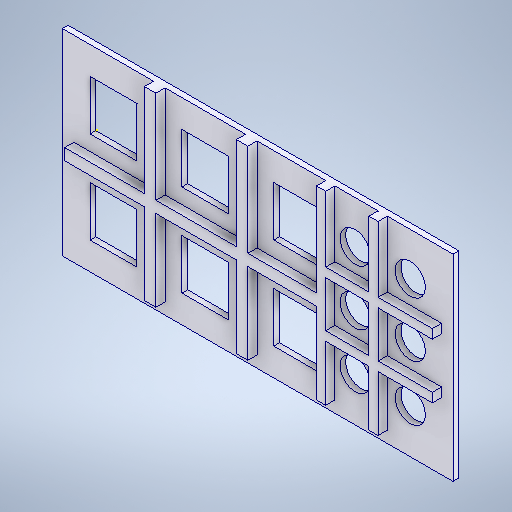
# Autodesk Inventor part: faceplate
Saved by Autodesk Inventor 2025 (Build 290162000, 162)
## iProperties
Created: 2024-08-10
Part Number: faceplate
Material: Generic
Document SubType Name: Modeling
Designer: ethan
Density: 1 g/cm^3
Appearance: Cool White
Author: ethan
Autodesk Inventor part; units mm, degrees
ref_plane "YZ Plane" through (0, 0, 0) normal (1, 0, 0) x (0, 1, 0)
ref_plane "XZ Plane" through (0, 0, 0) normal (0, 1, 0) x (-1, 0, 0)
ref_plane "XY Plane" through (0, 0, 0) normal (0, 0, 1) x (1, 0, 0)
sketch "Sketch1" plane through (0, 0, 0) normal (0, 0, 1) x (1, 0, 0)
  point P0 (0, 0)
sketch "Sketch2" plane through (0, 0, 0) normal (0, 0, 1) x (1, 0, 0)
  line L0 (0, 0) -> (20.4, 0)
  line L1 (20.4, 0) -> (20.4, 21.7)
  line L2 (20.4, 21.7) -> (0, 21.7)
  line L3 (0, 21.7) -> (0, 0)
  line L4 (40, 0) -> (60.4, 0)
  line L5 (60.4, 0) -> (60.4, 21.7)
  line L6 (60.4, 21.7) -> (40, 21.7)
  line L7 (40, 21.7) -> (40, 0)
  line L8 (80, 0) -> (100.4, 0)
  line L9 (100.4, 0) -> (100.4, 21.7)
  line L10 (100.4, 21.7) -> (80, 21.7)
  line L11 (80, 21.7) -> (80, 0)
  line L12 (0, -40) -> (20.4, -40)
  line L13 (20.4, -40) -> (20.4, -18.3)
  line L14 (20.4, -18.3) -> (0, -18.3)
  line L15 (0, -18.3) -> (0, -40)
  line L16 (40, -40) -> (60.4, -40)
  line L17 (60.4, -40) -> (60.4, -18.3)
  line L18 (60.4, -18.3) -> (40, -18.3)
  line L19 (40, -18.3) -> (40, -40)
  line L20 (80, -40) -> (100.4, -40)
  line L21 (100.4, -40) -> (100.4, -18.3)
  line L22 (100.4, -18.3) -> (80, -18.3)
  line L23 (80, -18.3) -> (80, -40)
  line L24 (100.4, 21.7) -> (175.4, 21.7) construction
  line L25 (175.4, 21.7) -> (175.4, -53.3) construction
  line L26 (175.4, -53.3) -> (100.4, -53.3) construction
  line L27 (100.4, -53.3) -> (100.4, 21.7) construction
  circle A0 centre (115.4, 15.1) radius 6.6 construction
  line L28 (115.4, 15.1) -> (115.4, -53.3) construction
  circle A1 centre (115.4, -8.9) radius 6.6 construction
  circle A2 centre (115.4, -32.9) radius 6.6 construction
  line L29 (100.4, 15.1) -> (200.3961, 15.1) construction
  circle A3 centre (139.4, 15.1) radius 6.6 construction
  circle A4 centre (139.4, -8.9) radius 6.6 construction
  circle A5 centre (139.4, -32.9) radius 6.6 construction
  circle A6 centre (115.4, 15.1) radius 6.6
  circle A7 centre (139.4, 15.1) radius 6.6 construction
  circle A8 centre (139.4, 15.1) radius 6.6
  circle A9 centre (115.4, -8.9) radius 6.6 construction
  circle A10 centre (115.4, -8.9) radius 6.6
  circle A11 centre (139.4, -8.9) radius 6.6 construction
  circle A12 centre (139.4, -8.9) radius 6.6
  circle A13 centre (115.4, -32.9) radius 6.6 construction
  circle A14 centre (115.4, -32.9) radius 6.6
  circle A15 centre (139.4, -32.9) radius 6.6 construction
  circle A16 centre (139.4, -32.9) radius 6.6
  line L30 (0, 21.7) -> (-12, 21.7) construction
  line L31 (-12, 21.7) -> (-12, 33.7) construction
  line L32 (-12, 33.7) -> (0, 33.7) construction
  line L33 (0, 33.7) -> (0, 21.7) construction
  line L34 (146, -40) -> (158, -40) construction
  line L35 (158, -40) -> (158, -52) construction
  line L36 (158, -52) -> (146, -52) construction
  line L37 (146, -52) -> (146, -40) construction
  line L38 (139.4, -32.9) -> (139.4, -74.4589) construction
  line L39 (-12, 33.7) -> (158, 33.7)
  line L40 (158, 33.7) -> (158, -52)
  line L41 (158, -52) -> (-12, -52)
  line L42 (-12, -52) -> (-12, 33.7)
  point P0 (146, -46)
  dimension "d0" = 20.4
  dimension "d1" = 21.7
  dimension "d5" = 40
  dimension "d8" = 40
  dimension "d11" = 75
  dimension "d12" = 75
  dimension "d13" = 13.2
  dimension "d14" = 15
  dimension "d15" = 13.2
  dimension "d16" = 24
  dimension "d17" = 13.2
  dimension "d18" = 24
  dimension "d19" = 61.7
  dimension "d20" = 13.2
  dimension "d21" = 24
  dimension "d22" = 13.2
  dimension "d23" = 13.2
  dimension "d26" = 24
  dimension "d29" = 24
  dimension "d32" = 12
  dimension "d33" = 12
  dimension "d34" = 12
  dimension "d35" = 12
  dimension "d36" = 6.6
  constraints: 86 end point, 17 centre point, 8 horizontal, 8 parallel, 7 perpendicular, 6 coincident, 5 point on line, 3 collinear, 3 vertical, 1 midpoint, 1 tangent, 58 other
  measures "d0" distance of L2.end L1.end
  measures "d1" distance of L0.end L1.end
  measures "d5" distance of L1.end L5.end
  measures "d8" distance of L1.end L13.end
  measures "d11" distance of L9.end L24.end
  measures "d12" distance of L24.end L25.end
  measures "d13" diameter of A0
  measures "d14" distance from line of L9 L28.start
  measures "d15" diameter of A1
  measures "d16" distance of A1.centre L28.start
  measures "d17" diameter of A2
  measures "d18" distance of A1.centre A2.centre
  measures "d19" distance between parallel lines of L20 L10
  measures "d20" diameter of A3
  measures "d21" distance of A3.centre L28.start
  measures "d22" diameter of A4
  measures "d23" diameter of A5
  measures "d26" distance of L28.start A7.centre
  measures "d29" distance of L28.start A9.centre
  measures "d32" distance of L31.end L32.end
  measures "d33" distance of L30.end L31.end
  measures "d34" distance of L35.end L36.end
  measures "d35" distance of L34.end L35.end
  measures "d36" distance from line of point (146, -46) L38
extrude "Extrusion1" add sketch "Sketch2" along normal blind 2.5
sketch "Sketch3" plane through (0, 0, 2.5) normal (0, 0, 1) x (1, 0, 0)
  line L0 (-12, -52) -> (158, -52) construction
  line L1 (158, -52) -> (158, 33.7) construction
  line L2 (158, 33.7) -> (-12, 33.7) construction
  line L3 (-12, 33.7) -> (-12, -52) construction
  circle A0 centre (115.4, 15.1) radius 6.6 construction
  circle A1 centre (139.4, 15.1) radius 6.6 construction
  circle A2 centre (115.4, -8.9) radius 6.6 construction
  circle A3 centre (139.4, -8.9) radius 6.6 construction
  circle A4 centre (115.4, -32.9) radius 6.6 construction
  circle A5 centre (139.4, -32.9) radius 6.6 construction
  line L4 (80, -40) -> (80, -18.3) construction
  line L5 (80, -18.3) -> (100.4, -18.3) construction
  line L6 (100.4, -18.3) -> (100.4, -40) construction
  line L7 (100.4, -40) -> (80, -40) construction
  line L8 (40, -40) -> (40, -18.3) construction
  line L9 (40, -18.3) -> (60.4, -18.3) construction
  line L10 (60.4, -18.3) -> (60.4, -40) construction
  line L11 (60.4, -40) -> (40, -40) construction
  line L12 (0, -40) -> (0, -18.3) construction
  line L13 (0, -18.3) -> (20.4, -18.3) construction
  line L14 (20.4, -18.3) -> (20.4, -40) construction
  line L15 (20.4, -40) -> (0, -40) construction
  line L16 (80, 0) -> (80, 21.7) construction
  line L17 (80, 21.7) -> (100.4, 21.7) construction
  line L18 (100.4, 21.7) -> (100.4, 0) construction
  line L19 (100.4, 0) -> (80, 0) construction
  line L20 (40, 0) -> (40, 21.7) construction
  line L21 (40, 21.7) -> (60.4, 21.7) construction
  line L22 (60.4, 21.7) -> (60.4, 0) construction
  line L23 (60.4, 0) -> (40, 0) construction
  line L24 (0, 0) -> (0, 21.7) construction
  line L25 (0, 21.7) -> (20.4, 21.7) construction
  line L26 (20.4, 21.7) -> (20.4, 0) construction
  line L27 (20.4, 0) -> (0, 0) construction
  line L28 (-7, 28.7) -> (153, 28.7) construction
  line L29 (153, 28.7) -> (153, -47) construction
  line L30 (153, -47) -> (-7, -47) construction
  line L31 (-7, -47) -> (-7, 28.7) construction
  line L32 (-7, -9.15) -> (-7, -6.65) construction
  line L33 (-7, -6.65) -> (-7, -11.65) construction
  line L34 (20.4, 21.7) -> (40, 21.7) construction
  line L35 (30.2, 21.7) -> (30.2, 28.7) construction
  line L36 (60.4, 21.7) -> (80, 21.7) construction
  line L37 (70.2, 21.7) -> (70.2, 28.7) construction
  line L38 (30.2, 28.7) -> (32.7, 28.7) construction
  line L39 (70.2, 28.7) -> (72.7, 28.7) construction
  line L40 (32.7, 28.7) -> (27.7, 28.7) construction
  line L41 (27.7, 28.7) -> (27.7, -47) construction
  line L42 (27.7, -47) -> (32.7, -47) construction
  line L43 (32.7, -47) -> (32.7, 28.7) construction
  line L44 (72.7, 28.7) -> (67.7, 28.7) construction
  line L45 (67.7, 28.7) -> (67.7, -47) construction
  line L46 (67.7, -47) -> (72.7, -47) construction
  line L47 (72.7, -47) -> (72.7, 28.7) construction
  circle A6 centre (115.4, 15.1) radius 6.6 construction
  line L48 (108.8, 15.1) -> (100.4, 15.1) construction
  line L49 (104.6, 15.1) -> (104.6, 28.7) construction
  line L50 (104.6, 28.7) -> (106.6, 28.7) construction
  line L51 (106.6, 28.7) -> (102.6, 28.7) construction
  line L52 (102.6, 28.7) -> (102.6, -47) construction
  line L53 (102.6, -47) -> (106.6, -47) construction
  line L54 (106.6, -47) -> (106.6, 28.7) construction
  line L55 (-7, -6.65) -> (-7, -11.65) construction
  line L56 (-7, -11.65) -> (106.6, -11.65) construction
  line L57 (106.6, -11.65) -> (106.6, -6.65) construction
  line L58 (106.6, -6.65) -> (-7, -6.65) construction
  line L59 (115.4, -2.3) -> (115.4, 8.5) construction
  line L60 (122, 15.1) -> (132.8, 15.1) construction
  line L61 (115.4, -26.3) -> (115.4, -15.5) construction
  line L62 (106.6, 3.1) -> (106.6, 1.1) construction
  line L63 (106.6, 1.1) -> (106.6, 5.1) construction
  line L64 (106.6, 5.1) -> (153, 5.1) construction
  line L65 (153, 5.1) -> (153, 1.1) construction
  line L66 (153, 1.1) -> (106.6, 1.1) construction
  line L67 (106.6, -20.9) -> (106.6, -22.9) construction
  line L68 (106.6, -22.9) -> (106.6, -18.9) construction
  line L69 (106.6, -18.9) -> (153, -18.9) construction
  line L70 (153, -18.9) -> (153, -22.9) construction
  line L71 (153, -22.9) -> (106.6, -22.9) construction
  line L72 (127.4, 28.7) -> (129.4, 28.7) construction
  line L73 (129.4, 28.7) -> (125.4, 28.7) construction
  line L74 (125.4, 28.7) -> (125.4, -47) construction
  line L75 (125.4, -47) -> (129.4, -47) construction
  line L76 (129.4, -47) -> (129.4, 28.7) construction
  line L77 (-7, -11.65) -> (106.6, -11.65)
  line L78 (106.6, -11.65) -> (106.6, -6.65)
  line L79 (106.6, -6.65) -> (-7, -6.65)
  line L80 (-7, -6.65) -> (-7, -11.65)
  line L81 (102.6, 28.7) -> (106.6, 28.7)
  line L82 (106.6, 28.7) -> (106.6, -47)
  line L83 (106.6, -47) -> (102.6, -47)
  line L84 (102.6, -47) -> (102.6, 28.7)
  line L85 (125.4, -47) -> (129.4, -47)
  line L86 (129.4, -47) -> (129.4, 28.7)
  line L87 (129.4, 28.7) -> (125.4, 28.7)
  line L88 (125.4, 28.7) -> (125.4, -47)
  line L89 (102.6, 5.1) -> (153, 5.1)
  line L90 (153, 5.1) -> (153, 1.1)
  line L91 (153, 1.1) -> (102.6, 1.1)
  line L92 (102.6, 1.1) -> (102.6, 5.1)
  line L93 (153, -18.9) -> (102.6, -18.9)
  line L94 (102.6, -18.9) -> (102.6, -22.9)
  line L95 (102.6, -22.9) -> (153, -22.9)
  line L96 (153, -22.9) -> (153, -18.9)
  line L97 (67.7, 28.7) -> (72.7, 28.7)
  line L98 (72.7, 28.7) -> (72.7, -47)
  line L99 (72.7, -47) -> (67.7, -47)
  line L100 (67.7, -47) -> (67.7, 28.7)
  line L101 (32.7, 28.7) -> (27.7, 28.7)
  line L102 (27.7, 28.7) -> (27.7, -47)
  line L103 (27.7, -47) -> (32.7, -47)
  line L104 (32.7, -47) -> (32.7, 28.7)
  line L105 (27.7, 28.7) -> (32.7, 28.7)
  line L106 (32.7, 28.7) -> (32.7, 33.7)
  line L107 (32.7, 33.7) -> (27.7, 33.7)
  line L108 (27.7, 33.7) -> (27.7, 28.7)
  line L109 (158, 33.7) -> (-12, 33.7) projected
  line L110 (67.7, 28.7) -> (72.7, 28.7)
  line L111 (72.7, 28.7) -> (72.7, 33.7)
  line L112 (72.7, 33.7) -> (67.7, 33.7)
  line L113 (67.7, 33.7) -> (67.7, 28.7)
  line L114 (102.6, 28.7) -> (106.6, 28.7)
  line L115 (106.6, 28.7) -> (106.6, 33.7)
  line L116 (106.6, 33.7) -> (102.6, 33.7)
  line L117 (102.6, 33.7) -> (102.6, 28.7)
  line L118 (125.4, 28.7) -> (129.4, 28.7)
  line L119 (129.4, 28.7) -> (129.4, 33.7)
  line L120 (129.4, 33.7) -> (125.4, 33.7)
  line L121 (125.4, 33.7) -> (125.4, 28.7)
  point P0 (102.6, -6.65)
  point P1 (72.7, -6.65)
  point P2 (67.7, -6.65)
  point P3 (32.7, -6.65)
  point P4 (27.7, -6.65)
  point P5 (27.7, -11.65)
  point P6 (32.7, -11.65)
  point P7 (67.7, -11.65)
  point P8 (72.7, -11.65)
  point P9 (102.6, -11.65)
  point P10 (125.4, -22.9)
  point P11 (129.4, -22.9)
  point P12 (129.4, -18.9)
  point P13 (129.4, 1.1)
  point P14 (129.4, 5.1)
  point P15 (125.4, 5.1)
  point P16 (106.6, 5.1)
  point P17 (125.4, 1.1)
  point P18 (125.4, -18.9)
  dimension "d39" = 5
  dimension "d40" = 2.5
  dimension "d42" = 2.5
  dimension "d43" = 2.5
  dimension "d44" = 5
  dimension "d45" = 5
  dimension "d46" = 2
  dimension "d47" = 4
  dimension "d48" = 5
  dimension "d49" = 2
  dimension "d50" = 4
  dimension "d51" = 2
  dimension "d52" = 4
  dimension "d53" = 2
  dimension "d54" = 4
  constraints: 184 end point, 36 parallel, 20 perpendicular, 17 point on line, 13 horizontal, 5 point on circle, 4 midpoint, 4 vertical, 1 collinear, 1 horizontal alignment, 1 vertical alignment, 20 other
  measures "d40" distance of L32.start L32.end
  measures "d42" distance of L35.end L38.end
  measures "d43" distance of L37.end L39.end
  measures "d44" distance of L38.end L40.end
  measures "d45" distance of L39.end L44.end
  measures "d46" distance of L49.end L50.end
  measures "d47" distance of L50.end L51.end
  measures "d48" distance of L32.end L33.end
  measures "d49" distance of L62.start L62.end
  measures "d50" distance of L62.end L63.end
  measures "d51" distance of L67.start L67.end
  measures "d52" distance of L67.end L68.end
  measures "d53" distance of L72.start L72.end
  measures "d54" distance of L72.end L73.end
extrude "Extrusion2" add sketch "Sketch3" along normal blind 4 contours L80 L79 L102 L77 | L102 L79 L104 L77 | L77 L104 L103 L102 | L104 L79 L100 L77 | L102 L101 L104 L79 | L100 L79 L98 L77 | L77 L98 L99 L100 | L108 L107 L106 L101 | L98 L79 L84 L77 | L100 L97 L98 L79 | L84 L79 L78 L77 | L77 L82 L93 L84 | L113 L109 L111 L97 | L93 L82 L95 L84 | L84 L91 L82 L79 | L93 L88 L95 L82 | L95 L82 L83 L84 | L84 L89 L82 L91 | L82 L89 L88 L91 | L93 L86 L95 L88 | L88 L91 L86 L93 | L84 L81 L82 L89 | L109 L115 L81 L117 | L88 L89 L86 L91 | L95 L86 L85 L88 | L93 L96 L95 L86 | L88 L87 L86 L89 | L86 L89 L90 L91 | L109 L119 L87 L121
body "Solid1"
